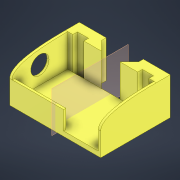
# Autodesk Inventor part: Electronics Tray
Saved by Autodesk Inventor 2022 (Build 260153000, 153)
## iProperties
Created: 2021-06-05
Part Number: Electronics Tray
Material: Generic
Document SubType Name: Modeling
Designer: sidsa
Density: 1 g/cm^3
Appearance: Smooth - Yellow
Author: sidsa
## iProperties of the stored document Electronics Tray_3DPrint.ipt
Created: 2021-06-06
Part Number: Electronics Tray_3DPrint
Material: Generic
Document SubType Name: Modeling
Designer: sidsa
Density: 1 g/cm^3
Appearance: Default
Author: sidsa
Autodesk Inventor part; units mm, degrees
ref_plane "YZ Plane" through (0, 0, 0) normal (1, 0, 0) x (0, 1, 0)
ref_plane "XZ Plane" through (0, 0, 0) normal (0, 1, 0) x (-1, 0, 0)
ref_plane "XY Plane" through (0, 0, 0) normal (0, 0, 1) x (1, 0, 0)
sketch "Sketch1" plane through (0, 0, 0) normal (0, 1, 0) x (-1, 0, 0)
  line L0 (-13.335, 9.525) -> (-18.415, 9.525)
  line L1 (-18.415, 9.525) -> (-18.415, 0)
  line L2 (-18.415, 0) -> (0, 0)
  line L3 (0, 3.175) -> (0, 0)
  line L4 (6.35, 9.525) -> (0, 3.175)
  line L5 (6.35, 9.525) -> (-5.715, 9.525)
  line L6 (-5.715, 6.35) -> (-5.715, 9.525)
  line L7 (-13.335, 6.35) -> (-5.715, 6.35)
  line L8 (-13.335, 9.525) -> (-13.335, 6.35)
  line L9 (25.4, 3.175) -> (19.05, 9.525)
  line L10 (25.4, 0) -> (25.4, 3.175)
  line L11 (25.4, 0) -> (43.815, 0)
  line L12 (43.815, 0) -> (43.815, 9.525)
  line L13 (43.815, 9.525) -> (38.735, 9.525)
  line L14 (38.735, 6.35) -> (38.735, 9.525)
  line L15 (31.115, 6.35) -> (38.735, 6.35)
  line L16 (31.115, 9.525) -> (31.115, 6.35)
  line L17 (31.115, 9.525) -> (19.05, 9.525)
  constraints: 36 end point
extrude "Extrusion1" add sketch "Sketch1" along normal blind 25.4
sketch "Sketch3" plane through (0, 0, 0) normal (0, -1, 0) x (1, 0, 0)
  line L0 (18.415, 9.525) -> (18.415, 0) projected
  line L1 (18.415, 9.525) -> (-43.815, 9.525)
  line L2 (-43.815, 9.525) -> (-43.815, 47.625)
  line L3 (-43.815, 47.625) -> (18.415, 47.625)
  line L4 (18.415, 47.625) -> (18.415, 9.525)
  line L5 (13.335, 9.525) -> (18.415, 9.525) projected
  line L6 (13.335, 9.525) -> (5.715, 9.525)
  line L7 (5.715, 9.525) -> (5.715, 9.652)
  line L8 (5.715, 9.652) -> (13.335, 9.652)
  line L9 (13.335, 9.652) -> (13.335, 9.525)
  line L10 (-31.115, 6.35) -> (-31.115, 9.525) projected
  line L11 (-31.115, 9.525) -> (-38.735, 9.525)
  line L12 (-38.735, 9.525) -> (-38.735, 9.652)
  line L13 (-38.735, 9.652) -> (-31.115, 9.652)
  line L14 (-31.115, 9.652) -> (-31.115, 9.525)
  point P0 (0, 0)
  dimension "d2" = 0.127
  dimension "d3" = 38.1
  constraints: 24 end point, 6 parallel, 3 horizontal, 3 perpendicular, 1 collinear
  measures "d2" distance between parallel lines of L1 L8
  measures "d3" distance between parallel lines of L3 L1
extrude "Extrusion2" add sketch "Sketch3" against normal blind 3.175 contours L1 L9 L8 L7 L14 L13 L12 L2 L3 L4
ref_plane "Work Plane1" through (-12.7, 0, 3.175) normal (1, 0, 0) x (0, 0, -1)
sketch "Sketch4" plane through (18.415, 0, 0) normal (1, 0, 0) x (0, 0, -1)
  line L0 (-47.625, 0) -> (-47.625, 3.175) projected
  line L1 (-9.525, 25.4) -> (-3.175, 25.4) projected
  line L2 (0, 0) -> (-47.625, 0) projected
  line L3 (0, 0) -> (0, 25.4) projected
  line L4 (-9.525, 25.4) -> (0, 25.4) projected
  line L5 (-9.525, 3.175) -> (-9.525, 25.4) projected
  line L6 (-47.625, 3.175) -> (-9.525, 3.175) projected
  line L7 (-47.625, 0) -> (-47.625, 3.175) projected
  line L8 (-9.525, 3.175) -> (-47.625, 3.175) projected
  line L9 (-47.625, 3.175) -> (-47.625, 15.875)
  line L10 (-9.525, 3.175) -> (-9.525, 25.4) projected
  line L11 (-9.525, 25.4) -> (-47.625, 25.4) construction
  line L12 (-47.625, 25.4) -> (-47.625, 15.875) construction
  spline S0 degree 2 poles (-9.525, 25.4) (-47.625, 25.4) (-47.625, 15.875) knots 1 1 1 2 2 2
  dimension "d6" = 12.7
  constraints: 2 end point, 1 perpendicular, 1 point on line, 1 vertical, 3 other
  measures "d6" distance of L0.end L9.end
extrude "Extrusion3" add sketch "Sketch4" against normal blind 1.5875 contours L9 S0 L5 L6
mirror "Mirror1" about plane through (-12.7, 0, 3.175) normal (1, 0, 0) of "Extrusion3"
sketch "Sketch5" plane through (0, 3.175, 0) normal (0, 1, 0) x (1, 0, 0)
  line L0 (-42.2275, -47.625) -> (16.8275, -47.625) projected
  line L1 (16.8275, -47.625) -> (-42.2275, -47.625)
  line L2 (-42.2275, -47.625) -> (-42.2275, -46.0375)
  line L3 (-42.2275, -46.0375) -> (16.8275, -46.0375)
  line L4 (16.8275, -46.0375) -> (16.8275, -47.625)
  point P0 (0, 0)
  dimension "d9" = 1.5875
  constraints: 8 end point, 2 parallel, 1 horizontal, 1 perpendicular
  measures "d9" distance between parallel lines of L0 L3
extrude "Extrusion4" add sketch "Sketch5" along normal blind 12.7
sketch "Sketch6" plane through (-43.815, 0, 47.625) normal (0, 0, 1) x (1, 0, 0)
  line L0 (60.6425, 15.875) -> (1.5875, 15.875) projected
  line L1 (60.6425, 15.875) -> (36.83, 15.875)
  line L2 (36.83, 15.875) -> (36.83, 3.175)
  line L3 (36.83, 3.175) -> (60.6425, 3.175)
  line L4 (60.6425, 3.175) -> (60.6425, 15.875)
  line L5 (62.23, 0) -> (0, 0) projected
  line L6 (62.23, 0) -> (62.23, 15.875) projected
  point P0 (43.815, 0)
  dimension "d12" = 3.175
  dimension "d13" = 25.4
  constraints: 8 end point, 2 parallel, 1 horizontal, 1 perpendicular
  measures "d12" distance between parallel lines of L5 L3
  measures "d13" distance between parallel lines of L6 L2
extrude "Extrusion5" cut sketch "Sketch6" against normal blind 12.7
sketch "Sketch7" plane through (-43.815, 0, 0) normal (-1, 0, 0) x (0, 0, 1)
  circle A0 centre (28.575, 15.24) radius 6.25
  line L0 (0, 25.4) -> (9.525, 25.4) projected
  line L1 (47.625, 0) -> (47.625, 15.875) projected
  point P0 (0, 0)
  dimension "d16" = 12.5
  dimension "d17" = 10.16
  dimension "d18" = 19.05
  constraints: 1 centre point
  measures "d16" diameter of A0
  measures "d17" distance from line of L0 A0.centre
  measures "d18" distance from line of L1 A0.centre
extrude "Extrusion6" cut sketch "Sketch7" against normal blind 12.7
chamfer "Chamfer1" distance 0.254 angle 45 1 edges at (-43.815, 15.24, 22.325)
body "Solid1"
